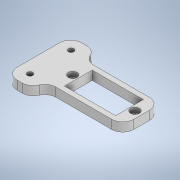
# Autodesk Inventor part: mount1
Saved by Autodesk Inventor 2020.2 (Build 242310000, 310)
## iProperties
Created: 2026-05-20
Part Number: mount1
Material: Generic
Document SubType Name: Modeling
Designer: explorer
Density: 1 g/cm^3
Appearance: Default
Author: explorer
Autodesk Inventor part; units mm, degrees
ref_plane "YZ Plane" through (0, 0, 0) normal (1, 0, 0) x (0, 1, 0)
ref_plane "XZ Plane" through (0, 0, 0) normal (0, 1, 0) x (-1, 0, 0)
ref_plane "XY Plane" through (0, 0, 0) normal (0, 0, 1) x (1, 0, 0)
sketch "Sketch1" plane through (0, 0, 0) normal (0, 1, 0) x (-1, 0, 0)
  line L0 (11.5, 6.25) -> (-11.5, 6.25)
  line L1 (-11.5, 6.25) -> (-11.5, -6.25)
  line L2 (-11.5, -6.25) -> (11.5, -6.25)
  line L3 (11.5, -6.25) -> (11.5, 6.25)
  line L4 (11.5, 6.25) -> (-11.5, -6.25) construction
  line L5 (-11.5, 6.25) -> (11.5, -6.25) construction
  line L6 (17, 8.5) -> (-17, 8.5)
  line L7 (-17, 8.5) -> (-17, -8.5)
  line L8 (-17, -8.5) -> (17, -8.5)
  line L9 (17, -8.5) -> (17, 8.5) construction
  line L10 (17, 8.5) -> (-17, -8.5) construction
  line L11 (-17, 8.5) -> (17, -8.5) construction
  line L12 (38.8, 0) -> (-26.3, 0) projected
  line L13 (0, -20.3) -> (0, 20.3) projected
  line L14 (29.5, 14.5) -> (18.5, 14.5)
  line L15 (18.5, 14.5) -> (18.5, -14.5) construction
  line L16 (18.5, -14.5) -> (29.5, -14.5)
  line L17 (29.5, -14.5) -> (29.5, 14.5)
  line L18 (29.5, 14.5) -> (18.5, -14.5) construction
  line L19 (18.5, 14.5) -> (29.5, -14.5) construction
  line L20 (18.5, 14.5) -> (17, 8.5)
  line L21 (17, -8.5) -> (18.5, -14.5)
  circle A0 centre (-14, 0) radius 1.15
  circle A1 centre (14, 0) radius 1.15
  circle A2 centre (24, 9.25) radius 1.25
  circle A3 centre (24, -9.25) radius 1.25
  point P0 (0, 0)
  point P1 (24, 0)
  dimension "d0" = 23
  dimension "d1" = 12.5
  dimension "d2" = 17
  dimension "d3" = 34
  dimension "d11" = 2.3
  dimension "d12" = 28
  dimension "d13" = 12.5
  dimension "d14" = 2.5
  dimension "d15" = 9.25
  dimension "d16" = 29
  dimension "d18" = 5.5
  constraints: 40 end point, 6 midpoint, 6 parallel, 4 centre point, 3 horizontal, 3 perpendicular, 2 point on line, 2 symmetric about line, 2 other
  measures "d0" distance of L1.end L2.end
  measures "d1" distance of L0.end L1.end
  measures "d2" distance of L6.end L7.end
  measures "d3" distance of L7.end L8.end
  measures "d11" diameter of A0
  measures "d12" distance of A0.centre A1.centre
  measures "d13" distance from line of L3 point (24, 0)
  measures "d14" diameter of A2
  measures "d15" distance of A2.centre point (24, 0)
  measures "d16" distance of L16.end L14.start
  measures "d18" distance from line of L17 point (24, 0)
extrude "Extrusion1" add sketch "Sketch1" along normal blind 4 contours L0 L13 L6 L20 L14 L17 L12 A1 L3 | L0 L1 L12 A0 L7 L6 L13 | L12 A1 L17 L16 L21 L8 L13 L2 L3 | L1 L2 L13 L8 L7 L12 A0
sketch "Sketch2" plane through (0, 4, 0) normal (0, 1, 0) x (1, 0, 0)
  circle A0 centre (14, 0) radius 1.15 projected
  circle A1 centre (14, 0) radius 2
  line L0 (0, 20.3) -> (0, -20.3) projected
  circle A2 centre (-14, 0) radius 2
  point P0 (0, 0)
  dimension "d21" = 4
  constraints: 2 centre point, 1 coincident, 1 symmetric about line, 1 other
  measures "d21" diameter of A1
extrude "Extrusion2" cut sketch "Sketch2" against normal blind 2
sketch "Sketch3" plane through (0, 0, 0) normal (0, -1, 0) x (1, 0, 0)
  line L0 (-38.8, 0) -> (26.3, 0) projected
  circle A0 centre (-24, 9.25) radius 1.25 projected
  circle A1 centre (-24, 9.25) radius 2.25
  circle A2 centre (-24, -9.25) radius 2.25
  point P0 (0, 0)
  dimension "d24" = 4.5
  constraints: 2 centre point, 1 coincident, 1 symmetric about line, 1 other
  measures "d24" diameter of A1
extrude "Extrusion3" cut sketch "Sketch3" against normal blind 2 contours A0 | A1 | A2
fillet "Fillet1" radius 5 8 edges at (-18.5, 2, 14.5) (-17, 2, 8.5) (-29.5, 2, 14.5) (-29.5, 2, -14.5) (-18.5, 2, -14.5) (-17, 2, -8.5) (17, 2, -8.5) (17, 2, 8.5)
body "Solid1"
